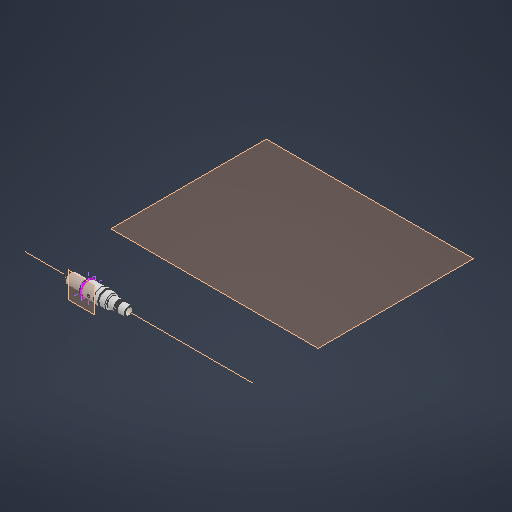
# Autodesk Inventor part: nakrętka otwor w pionie
Saved by Autodesk Inventor 2026.1 (Build 301233020, 233B)
## iProperties
Created: 2026-02-26
Part Number: nakrętka otwor w pionie
Material: Generic
Document SubType Name: Modeling
Designer: Jan
Density: 1 g/cm^3
Appearance: Default
Author: Jan
Autodesk Inventor part; units mm, degrees
ref_plane "YZ Plane" through (0, 0, 0) normal (1, 0, 0) x (0, 1, 0)
ref_plane "XZ Plane" through (0, 0, 0) normal (0, 1, 0) x (-1, 0, 0)
ref_plane "XY Plane" through (0, 0, 0) normal (0, 0, 1) x (1, 0, 0)
sketch "Sketch2" plane through (0, 0, 0) normal (0, 0, 1) x (1, 0, 0)
  line L0 (0, 4) -> (0.5, 4.5)
  line L1 (0, 4) -> (0, 3)
  line L2 (0.5, 4.5) -> (1.1, 4.5)
  line L3 (1.1, 4.5) -> (1.1, 4.3)
  line L4 (1.1, 4.3) -> (2.1, 4.3)
  line L5 (2.1, 4.3) -> (2.1, 4.5)
  line L6 (2.1, 4.5) -> (14.8, 4.5)
  line L7 (15.1, 4.5) -> (15.1, 5.5)
  line L8 (15.1, 5.5) -> (15.6, 6)
  line L9 (44.15, 4.5) -> (44.15, 4.3)
  line L10 (44.15, 4.3) -> (43.15, 4.3)
  line L11 (43.15, 4.3) -> (43.15, 4.5)
  line L12 (0, 0) -> (27.0854, 0) construction
  line L13 (15.6, 6) -> (16.1, 6)
  line L14 (16.1, 6) -> (16.1, 5)
  line L15 (16.1, 5) -> (17.1, 5)
  line L16 (17.1, 5) -> (17.1, 6)
  line L17 (31.9, 6) -> (31.8, 6)
  line L18 (31.5, 6) -> (31.5, 6.5)
  line L19 (31.5, 6.5) -> (28.1, 6.5)
  line L20 (28.1, 6.5) -> (28.1, 6)
  line L21 (17.1, 6) -> (28.1, 6)
  line L22 (21, 3.2) -> (43.9, 3.2)
  line L23 (44.15, 4.5) -> (45.15, 4.5)
  line L24 (43.15, 4.5) -> (37.9, 4.5)
  line L25 (37.15, 6) -> (31.9, 6)
  line L26 (43.9, 3.2) -> (49.9, 3.2)
  line L27 (49.9, 4) -> (45.45, 4)
  line L28 (45.15, 4) -> (45.15, 4.5)
  line L29 (49.9, 3.2) -> (51.9, 3.2)
  line L30 (51.9, 3.2) -> (51.9, 4)
  line L31 (51.9, 4) -> (49.9, 4)
  line L32 (37.9, 4.5) -> (37.45, 4.5)
  line L33 (37.15, 4.5) -> (37.15, 6)
  line L34 (15.1, 4.5) -> (15.1, 4.3)
  line L35 (15.1, 4.3) -> (14.8, 4.3)
  line L36 (14.8, 4.3) -> (14.8, 4.5)
  line L37 (31.5, 6) -> (31.5, 5.8)
  line L38 (31.5, 5.8) -> (31.8, 5.8)
  line L39 (31.8, 5.8) -> (31.8, 6)
  line L40 (37.15, 4.5) -> (37.15, 4.3)
  line L41 (37.15, 4.3) -> (37.45, 4.3)
  line L42 (37.45, 4.3) -> (37.45, 4.5)
  line L43 (45.15, 4) -> (45.15, 3.8)
  line L44 (45.15, 3.8) -> (45.45, 3.8)
  line L45 (45.45, 3.8) -> (45.45, 4)
  line L46 (0, 3) -> (0, 0)
  line L47 (0, 0) -> (20, 0)
  line L48 (20, 2.2) -> (20, 0)
  line L49 (20, 2.2) -> (21, 3.2)
  point P0 (1.1, 4.4)
  point P1 (15.85, 6)
  point P2 (16.6, 5)
  dimension "d3" = 4
  dimension "d8" = 1
  dimension "d9" = 0.5
  dimension "d10" = 0.5
  dimension "d11" = 0.2
  dimension "d12" = 1
  dimension "d13" = 13
  dimension "d14" = 1
  dimension "d29" = 0.5
  dimension "d30" = 0.5
  dimension "d36" = 1.1
  dimension "d37" = 4.5
  dimension "d38" = 3
  dimension "d39" = 0.5
  dimension "d40" = 1
  dimension "d41" = 1
  dimension "d60" = 0.4
  dimension "d61" = 0.5
  dimension "d62" = 3.4
  dimension "d63" = 11
  dimension "d65" = 1
  dimension "d66" = 5.25
  dimension "d83" = 6
  dimension "d84" = 0.8
  dimension "d85" = 2
  dimension "d86" = 0.75
  dimension "d105" = 0.2
  dimension "d106" = 0.3
  dimension "d107" = 0.2
  dimension "d108" = 0.3
  dimension "d109" = 0.2
  dimension "d110" = 0.3
  dimension "d111" = 0.2
  dimension "d112" = 0.3
  constraints: 100 end point, 19 perpendicular, 16 horizontal, 6 vertical, 3 midpoint, 1 point on line
  measures "d3" distance of L12.start L0.start
  measures "d8" distance of L0.start L1.end
  measures "d9" horizontal distance of L0.end L0.start
  measures "d10" horizontal distance of L0.end L0.start
  measures "d11" distance of L2.end L3.end
  measures "d12" distance of L3.end L4.end
  measures "d13" distance of L5.end L7.start
  measures "d14" distance of L7.start L7.end
  measures "d29" horizontal distance of L8.end L7.end
  measures "d30" horizontal distance of L8.end L7.end
  measures "d36" horizontal distance of point (1.1, 4.4) L12.start
  measures "d37" distance from line of L6 L12.start
  measures "d38" distance of L1.end L12.start
  measures "d39" distance of L8.end L13.end
  measures "d40" distance of L14.end L15.end
  measures "d41" vertical distance of point (15.85, 6) point (16.6, 5)
  measures "d60" distance of L17.start L18.start
  measures "d61" distance of L18.start L18.end
  measures "d62" distance of L18.end L19.end
  measures "d63" distance of L16.end L20.end
  measures "d65" distance of L9.start L23.end
  measures "d66" distance of L11.end L24.end
  measures "d83" distance of L22.end L26.end
  measures "d84" distance of L26.end L27.start
  measures "d85" distance of L26.end L29.end
  measures "d86" distance of L24.end L33.start
  measures "d105" distance of L7.start L34.end
  measures "d106" distance of L34.end L35.end
  measures "d107" distance of L18.start L37.end
  measures "d108" distance of L37.end L38.end
  measures "d109" distance of L33.start L40.end
  measures "d110" distance of L40.end L41.end
  measures "d111" distance of L28.start L43.end
  measures "d112" distance of L43.end L44.end
revolve "Revolution1" add sketch "Sketch2" angle 360 about axis through (0, 0, 0) along (1, 0, 0)
thread "Thread1" size "M6x1" class "6H" standard "ISO Metric profile" full length
ref_plane "Work Plane1" through (51.1424, -20, -139.2633) normal (0, 1, 0) x (-1, 0, 0)
sketch "Sketch4" plane through (17.1, 0, 0) normal (-1, 0, 0) x (0, 0, 1)
  circle A0 centre (0, 0) radius 6 projected
  point P0 (0, 6)
  point P1 (6, 0)
  point P2 (0, -6.0107)
  point P3 (-6.0435, 0)
  constraints: 2 point on circle
chamfer "Chamfer3" distance 0.3 angle 45 1 edges at (51.9, -4, 0)
ref_plane "Work Plane4" through (17.1, 0, 6) normal (0, 0, 1) x (1, 0, 0)
sketch "Sketch8" plane through (17.1, 0, 6) normal (0, 0, 1) x (1, 0, 0)
  circle A0 centre (6.1, 0) radius 1
  line L0 (0, -6) -> (0, 6) projected
  point P0 (-17.1, 0)
  dimension "d90" = 2
  dimension "d91" = 6.1
  constraints: 1 centre point
  measures "d90" diameter of A0
  measures "d91" distance from line of A0.centre L0
hole "Hole3" at (23.2, 0, 6) direction (0, 0, -1) diameter 1.567 depth 6.3 tip angle 118 thread size "M2x0.4" class "6H" standard "ISO Metric profile"
chamfer "Chamfer4" distance 0.2 angle 45 3 edges at (22.6668, -0.5741, 5.9725) (23.7332, -0.5741, 5.9725) (23.2, 0.7835, 5.9486)
chamfer "Chamfer5" distance 0.3 angle 45 1 edges at (51.9, -3.2, 0)
sketch "Sketch9" plane through (0, 0, 0) normal (-1, 0, 0) x (0, 0, 1)
  circle A0 centre (0, 0) radius 1.2953
  constraints: 1 centre point, 1 coincident
hole "Hole4" at (0, 0, 0) direction (1, 0, 0) diameter 4.917 end through all thread size "M6x1" class "6H" standard "ISO Metric profile"
chamfer "Chamfer6" distance 0.5 angle 45 1 edges at (0, 0, -2.4585)
body "Solid2"
